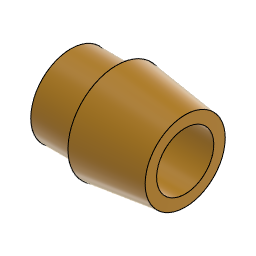
Barbed_Cover (Autodesk Fusion 360 design; units mm, degrees)
Autodesk Fusion 360 part; units mm, degrees
sketch "Sketch1" plane through (0, 0, 0) normal (0, 1, 0) x (1, 0, 0)
  line L0 (0, 0) -> (6, 0)
  line L1 (6, 0) -> (6, -1.5)
  line L2 (6, -1.5) -> (0, -1.5)
  line L3 (0, -1.5) -> (0, 0)
  line L4 (0, 0) -> (6, 0)
  line L5 (6, 0) -> (6, -2.1)
  line L6 (6, -2.1) -> (0, -2.1)
  line L7 (0, -2.1) -> (0, 0)
  line L8 (6, -2.1) -> (2.4, -2.1)
  line L9 (2.4, -2.1) -> (2.4, -2.55)
  line L10 (2.4, -2.55) -> (6, -2.1)
  dimension "d4" = 6
  dimension "d5" = 1.5
  dimension "d6" = 6
  dimension "d7" = 2.1
  dimension "d11" = 3.6
  dimension "d12" = 0.45
  constraint horizontal L0
  constraint vertical L1
  constraint horizontal L2
  constraint vertical L3
  constraint coincident L0.start L3.end
  constraint horizontal L4
  constraint vertical L5
  constraint horizontal L6
  constraint vertical L7
  constraint perpendicular L5 L8
  constraint perpendicular L6 L9
  measures "d4" distance of L0.start L0.end
  measures "d5" distance of L0.start L2.end
  measures "d6" distance of L0.start L0.end
  measures "d7" distance of L0.start L6.end
  measures "d11" distance of L5.end L8.end
  measures "d12" distance of L8.end L9.end
revolve "Revolve1" add sketch "Sketch1" angle 360 about axis through (0, 0, 0) along (1, 0, 0) contours L2 L5 L6 L7 L8 | L6 L8 L9 L10
equation "Barbless_OD = 3 mm"
equation "minWallThickness = 0.6 mm"
equation "Barbless_Length = 6 mm"
equation "d4 = Barbless_Length"
equation "d5 = Barbless_OD / 2"
equation "d6 = Barbless_Length"
equation "d7 = Barbless_OD / 2 + minWallThickness"
equation "Barb_FLength = 3.6 mm"
equation "Barb_FD = 4.5 mm"
equation "Barb_FE = Barb_FD - ( Barbless_Length / 2 + minWallThickness )"
equation "d11 = Barb_FLength"
equation "d12 = Barb_FE / 2"
